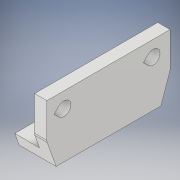
# Autodesk Inventor part: Y-axis Belt Idler 1
Saved by Autodesk Inventor 2018 (Build 220112000, 112)
## iProperties
Created: 2013-10-27
Part Number: Y-axis Belt Idler 1
Material: ASA Plastic
Document SubType Name: Modeling
Designer: Gabriel Smolnycki
Mass: 4.57544 g
Surface Area: 28.6329 cm^2
Volume: 4.27611 cm^3
Density: 1.07 g/cm^3
Appearance: Smooth - White ASA
Sending System: SolidWorks 2017
Last Author: Gabriel Smolnycki
Last Saved: 2017-09-14
Author: Gabriel Smolnycki
Autodesk Inventor part; units mm, degrees
ref_plane "YZ Plane" through (0, 0, 0) normal (1, 0, 0) x (0, 1, 0)
ref_plane "XZ Plane" through (0, 0, 0) normal (0, 1, 0) x (-1, 0, 0)
ref_plane "XY Plane" through (0, 0, 0) normal (0, 0, 1) x (1, 0, 0)
sketch "Sketch1" plane through (0, 0, 0) normal (0, 0, 1) x (1, 0, 0)
  line L0 (-3, 0) -> (-3, 20)
  line L1 (-15, 0) -> (-3, 0)
  line L2 (-15, 4) -> (-15, 0)
  line L3 (-7, 4) -> (-15, 4)
  line L4 (-7, 20) -> (-7, 4)
  line L5 (-3, 20) -> (-7, 20)
  constraints: 12 end point, 3 horizontal, 3 vertical, 1 perpendicular
extrude "Extrusion4" add sketch "Sketch1" along normal blind 40
sketch "Sketch2" plane through (-15, 4, 0) normal (0, 1, 0) x (1, 0, 0)
  arc A0 (5.591, -13.591) -> (2.409, -13.591) centre (4, -12) ccw
  line L0 (4, -15.182) -> (5.591, -13.591)
  line L1 (2.409, -13.591) -> (4, -15.182)
  line L2 (8, 0) -> (0, 0) projected
  line L3 (0, 0) -> (0, -40) projected
  arc A1 (5.591, -29.591) -> (2.409, -29.591) centre (4, -28) ccw
  line L4 (4, -31.182) -> (5.591, -29.591)
  line L5 (2.409, -29.591) -> (4, -31.182)
  line L6 (8, -40) -> (0, -40) projected
  dimension "d8" = 2.25
  dimension "d9" = 12
  dimension "d10" = 4
  dimension "d11" = 2.25
  dimension "d12" = 2.25
  dimension "d13" = 2.25
  dimension "d14" = 12
  dimension "d15" = 4
  constraints: 8 end point, 4 perpendicular, 4 point on circle, 2 centre point, 2 vertical alignment
  measures "d8" radius of A0
  measures "d9" distance from line of A0.centre L2
  measures "d10" distance from line of L3 A0.centre
  measures "d11" distance of L1.start L0.start
  measures "d12" radius of A1
  measures "d13" distance of L5.start L4.start
  measures "d14" distance from line of L6 A1.centre
  measures "d15" distance from line of L3 A1.centre
extrude "Extrusion3" cut sketch "Sketch2" against normal blind 4
sketch "Sketch3" plane through (-7, 4, 0) normal (-1, 0, 0) x (0, 0, 1)
  arc A0 (7.091, 12.591) -> (7.091, 9.409) centre (5.5, 11) ccw
  line L0 (8.682, 11) -> (7.091, 9.409)
  line L1 (7.091, 12.591) -> (8.682, 11)
  constraints: 4 end point, 2 perpendicular, 2 point on circle, 1 centre point
extrude "Extrusion2" cut sketch "Sketch3" against normal blind 4 draft 0
sketch "Sketch4" plane through (-7, 4, 0) normal (-1, 0, 0) x (0, 0, 1)
  arc A0 (36.091, 12.591) -> (36.091, 9.409) centre (34.5, 11) ccw
  line L0 (37.682, 11) -> (36.091, 9.409)
  line L1 (36.091, 12.591) -> (37.682, 11)
  constraints: 4 end point, 2 perpendicular, 2 point on circle, 1 centre point
extrude "Extrusion1" cut sketch "Sketch4" against normal blind 4 draft 0
sketch "Sketch5" plane through (-3, 0, 0) normal (1, 0, 0) x (0, 0, -1)
  arc A0 (-36.091, 13.409) -> (-36.091, 16.591) centre (-34.5, 15) ccw projected
  line L0 (-40, 0) -> (-40, 20) projected
  circle A1 centre (-34.5, 15) radius 6.5 construction
  line L1 (0, 0) -> (-40, 0) projected
  line L2 (-37, 0) -> (-39.886, 8.1769)
  arc A2 (-40, 8.8426) -> (-39.886, 8.1769) centre (-38, 8.8426) ccw
  line L3 (-37, 0) -> (-40, 0)
  line L4 (-40, 0) -> (-40, 8.8426)
  line L5 (-20, 22.0768) -> (-20, -2.8383) construction
  line L6 (-3, 0) -> (-0.114, 8.1769)
  arc A3 (-0.114, 8.1769) -> (0, 8.8426) centre (-2, 8.8426) ccw
  line L7 (-3, 0) -> (0, 0)
  line L8 (0, 0) -> (0, 8.8426)
  point P0 (-40, 8.5)
  dimension "d16" = 13
  dimension "d17" = 3
  dimension "d18" = 6.5
  dimension "d19" = 2
  constraints: 14 end point, 4 point on circle, 4 symmetric about line, 3 centre point, 3 point on line, 1 coincident, 1 collinear, 1 horizontal alignment, 1 perpendicular, 1 tangent, 1 vertical, 1 other
  measures "d16" diameter of A1
  measures "d17" distance of L0.start L2.start
  measures "d18" vertical distance of point (-40, 8.5) A0.centre
  measures "d19" radius of A2
extrude "Extrusion7" cut sketch "Sketch5" against normal through all
body "Solid3"
